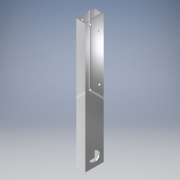
# Autodesk Inventor part: 15102898-16-A-0301
Saved by Autodesk Inventor 2017 (Build 210142000, 142)
## iProperties
Created: 2016-10-02
Part Number: 15102898-16-A-0301
Material: Aluminum 6061
Document SubType Name: Sheet Metal
Designer: gus
Density: 2.7 g/cm^3
Appearance: Aluminum - Flat
Sheet Metal Rule: Default
Author: gus
Autodesk Inventor part; units mm, degrees
ref_plane "YZ Plane" through (0, 0, 0) normal (1, 0, 0) x (0, 1, 0)
ref_plane "XZ Plane" through (0, 0, 0) normal (0, 1, 0) x (-1, 0, 0)
ref_plane "XY Plane" through (0, 0, 0) normal (0, 0, 1) x (1, 0, 0)
sketch "Sketch1" plane through (0, 0, 0) normal (0, 1, 0) x (-1, 0, 0)
  line L0 (0, 0) -> (-25.4, 0)
  line L1 (-25.4, 0) -> (-25.4, 50.8)
  line L2 (-25.4, 50.8) -> (0, 50.8)
  line L3 (0, 50.8) -> (0, 0)
  line L4 (-3.175, 3.175) -> (-22.225, 3.175)
  line L5 (-22.225, 3.175) -> (-22.225, 47.625)
  line L6 (-22.225, 47.625) -> (-3.175, 47.625)
  line L7 (-3.175, 47.625) -> (-3.175, 3.175)
  dimension "d0" = 25.4
  dimension "d1" = 50.8
  dimension "d2" = 3.175
  constraints: 16 end point, 4 parallel, 2 perpendicular, 1 horizontal, 3 other
  measures "d0" distance of L1.end L2.end
  measures "d1" distance of L0.end L1.end
  measures "d2" distance between parallel lines of L3 L7
extrude "Extrusion1" add sketch "Sketch1" along normal blind 355.6
sketch "Sketch2" plane through (25.4, 0, 50.8) normal (1, 0, 0) x (0, 0, -1)
  circle A0 centre (25.4, 25.4) radius 14.2875
  line L0 (50.8, 0) -> (50.8, 355.6) projected
  line L1 (50.8, 0) -> (0, 0) projected
  dimension "d5" = 28.575
  dimension "d6" = 25.4
  dimension "d7" = 25.4
  constraints: 1 centre point
  measures "d5" diameter of A0
  measures "d6" distance from line of L0 A0.centre
  measures "d7" distance from line of L1 A0.centre
extrude "Extrusion2" cut sketch "Sketch2" against normal blind 25.4
sketch "Sketch3" plane through (0, 0, 0) normal (-1, 0, 0) x (0, 0, 1)
  line L0 (50.8, 0) -> (50.8, 355.6) projected
  line L1 (0, 355.6) -> (50.8, 355.6) projected
  line L2 (0, 0) -> (0, 355.6) projected
  line L3 (0, 0) -> (50.8, 0) projected
  point P0 (38.1, 346.075)
  point P1 (38.1, 190.5)
  point P2 (38.1, 320.675)
  point P3 (12.7, 215.9)
  dimension "d10" = 12.7
  dimension "d11" = 9.525
  dimension "d19" = 25.4
  dimension "d20" = 38.1
  dimension "d21" = 38.1
  dimension "d23" = 190.5
  dimension "d26" = 215.9
  dimension "d27" = 12.7
  measures "d10" distance from line of L0 point (38.1, 346.075)
  measures "d11" distance from line of L1 point (38.1, 346.075)
  measures "d19" distance of point (38.1, 346.075) point (38.1, 320.675)
  measures "d20" distance from line of L2 point (38.1, 320.675)
  measures "d21" distance from line of L2 point (38.1, 190.5)
  measures "d23" distance from line of L3 point (38.1, 190.5)
  measures "d26" distance from line of L3 point (12.7, 215.9)
  measures "d27" distance from line of point (12.7, 215.9) L2
hole "Hole1" at (0, 346.075, 38.1) at (0, 320.675, 38.1) at (0, 190.5, 38.1) at (0, 215.9, 12.7) direction (1, 0, 0) diameter 6.35 end through all
equation "\"BendRadius\" = Thickness"
equation "\"BendReliefWidth\" = Thickness"
equation "\"BendReliefDepth\" = 0.5 * Thickness"
equation "\"CornerReliefSize\" = 4 * Thickness"
equation "\"MinimumRemnant\" = 2 * Thickness"
equation "\"TransitionRadius\" = BendRadius"
equation "\"JacobiRadiusSize\" = Thickness"
equation "\"GapSize\" = Thickness"
equation "\"Thickness\" = 3.048"
body "Solid1"
